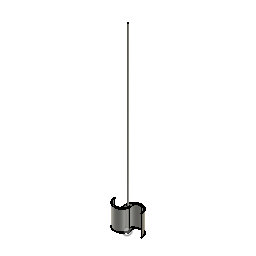
Savonius Turbine (Autodesk Fusion 360 design; units mm, degrees)
Autodesk Fusion 360 part; units mm, degrees
note: some values were not read from the file. Set by a fixed rule: which face or edge a step refers to.
sketch "Turbine Blade" plane through (0, 0, 0) normal (0, 0, 1) x (1, 0, 0) in component "Savonius Turbine"
  circle A0 centre (0, 0) radius 10.5 construction
  line L0 (0, 0) -> (-10.5, 0) construction
  line L1 (-10.5, 0) -> (75, 0) construction
  arc A1 (75, 0) -> (-10.5, 0) centre (32.25, 0) ccw
  arc A2 (74.2, 0) -> (-9.7, 0) centre (32.25, 0) ccw
  line L2 (74.2, 0) -> (75, 0)
  line L3 (-10.5, 0) -> (-9.7, 0) construction
  line L4 (-9.7, 0) -> (-10.5, 0)
  line L5 (75, 0) -> (37.5, 0)
  arc A3 (74.2, 0) -> (37.5, 36.7) centre (37.5, 0) ccw
  line L6 (37.5, 0) -> (74.2, 0) construction
  line L7 (37.5, 0) -> (37.5, 36.7) construction
  line L8 (37.5, 36.7) -> (0, 36.7) construction
  line L9 (0, 36.7) -> (-9.7, 0) construction
  spline S0 degree 2 poles (37.5, 36.7) (0, 36.7) (-9.7, 0) knots 0 0 0 1 1 1
  dimension "d57" = 21
  dimension "d59" = 75
  dimension "d84" = 42.75
  dimension "d87" = 37.5
  dimension "d88" = 90
  constraint coincident A0.centre L0.start
  constraint coincident A0 L0.end
  constraint horizontal L0
  constraint horizontal L1
  constraint parallel L1 L2
  constraint parallel L1 L3
  constraint coincident L1 L5.end
  constraint coincident L5.end A3.centre
  constraint horizontal L8
  constraint vertical A0.centre L8.end
  measures "d57" diameter of A0
  measures "d59" distance of L1.end A0.centre
  measures "d84" radius of A1
  measures "d87" distance of L1.end L5.end
  measures "d88" angle of L6 L7
extrude "Extrude5" add sketch "Turbine Blade" along normal blind 115.5 makes body 1 in component "Savonius Turbine"
pattern_circular "C-Pattern1" count 2 over 360 about axis through (0, 0, 1.75) along (0, 0, 1) of bodies 1 makes body 2 in component "Savonius Turbine"
sketch "EndPlates" plane through (0, 0, 0) normal (0, 0, 1) x (1, 0, 0) in component "Savonius Turbine"
  circle A0 centre (0, 0) radius 82.5
  line L0 (7.4921, 18.5437) -> (-7.4921, -18.5437) construction
  circle A1 centre (7.4921, 18.5437) radius 1.5
  circle A2 centre (-7.4921, -18.5437) radius 1.5
  line L1 (20, 0) -> (2.5, 0)
  circle A3 centre (0, 0) radius 4.25
  arc A4 (75, 0) -> (-10.5, 0) centre (32.25, 0) ccw
  line L2 (-10.5, 0) -> (-9.7, 0)
  spline S0 degree 2 poles (-9.7, 0) (0, 36.7) (37.5, 36.7) knots -1 -1 -1 0 0 0
  arc A5 (74.2, 0) -> (37.5, 36.7) centre (37.5, 0) ccw
  line L3 (74.2, 0) -> (75, 0)
  arc A6 (-75, 0) -> (10.5, 0) centre (-32.25, 0) ccw
  line L4 (10.5, 0) -> (9.7, 0)
  spline S1 degree 2 poles (9.7, 0) (0, -36.7) (-37.5, -36.7) knots -1 -1 -1 0 0 0
  arc A7 (-74.2, 0) -> (-37.5, -36.7) centre (-37.5, 0) ccw
  line L5 (-74.2, 0) -> (-75, 0)
  arc A8 (-72.1423, 2) -> (-37.5, -34.7) centre (-37.5, 0) ccw
  spline S2 degree 3 poles (8.1599, 2) (8.0288, 1.5037) (7.8976, 1.0074) (7.7664, 0.5111) (4.8101, -10.674) (-0.0689, -19.0509) (-6.813, -24.8318) (-13.502, -30.5653) (-22.0851, -33.8174) (-32.8116, -34.5451) (-34.332, -34.6482) (-35.8948, -34.7) (-37.5, -34.7) knots -1.020285 -1.020285 -1.020285 -1.020285 -1 -1 -1 -0.531046 -0.531046 -0.531046 -0.065928 -0.065928 -0.065928 0 0 0 0
  line L6 (12.4553, 2) -> (8.1599, 2)
  arc A9 (-76.9553, 2) -> (12.4553, 2) centre (-32.25, 0) ccw
  line L7 (-72.1423, 2) -> (-76.9553, 2)
  arc A10 (72.1423, -2) -> (37.5, 34.7) centre (37.5, 0) ccw
  spline S3 degree 3 poles (-8.1599, -2) (-8.0288, -1.5037) (-7.8976, -1.0074) (-7.7664, -0.5111) (-4.8101, 10.674) (0.0689, 19.0509) (6.813, 24.8318) (13.502, 30.5653) (22.0851, 33.8174) (32.8116, 34.5451) (34.332, 34.6482) (35.8948, 34.7) (37.5, 34.7) knots -1.020285 -1.020285 -1.020285 -1.020285 -1 -1 -1 -0.531046 -0.531046 -0.531046 -0.065928 -0.065928 -0.065928 0 0 0 0
  line L8 (-12.4553, -2) -> (-8.1599, -2)
  arc A11 (76.9553, -2) -> (-12.4553, -2) centre (32.25, 0) ccw
  line L9 (72.1423, -2) -> (76.9553, -2)
  line L10 (-12.4553, -2) -> (-11.2868, -28.1194)
  line L11 (12.4553, 2) -> (11.2868, 28.1194)
  dimension "d65" = 165
  dimension "d68" = 40
  dimension "d69" = 3
  dimension "d70" = 3
  dimension "d71" = 68
  dimension "d72" = 8.5
  dimension "d89" = 2
  dimension "d90" = 2
  constraint coincident A0.centre A3.centre
  constraint midpoint L0 A0.centre
  constraint coincident L0.start A1.centre
  constraint coincident L0.end A2.centre
  constraint concentric A0 A3
  constraint coincident S2 L10.end
  constraint tangent A11 L10
  constraint coincident S3 L11.end
  constraint tangent A9 L11
  measures "d65" diameter of A0
  measures "d68" distance of L0.start L0.end
  measures "d69" diameter of A1
  measures "d70" diameter of A2
  measures "d71" angle of L0 L1
  measures "d72" diameter of A3
extrude "Extrude6" add sketch "EndPlates" along normal blind 2.4 separate body contours L1 A6 L4 S1 A7 L5 | L1 L4 S2 L6 A9 | L1 A6 S1 A7 L5 A8 S2 A9 L7 | S2 L6 S3 L8 L10 L11 | A10 S3 L8 A11 L9 | A4 L2 S0 A5 L3 makes body 3 in component "Savonius Turbine"
extrude "Extrude7" add sketch "EndPlates" along normal mid plane 2.4 from surface at 115.5 separate body contours L1 A6 L4 S1 A7 L5 | L1 L4 S2 L6 A9 | L1 A6 S1 A7 L5 A8 S2 A9 L7 | S2 L6 S3 L8 L10 L11 | A10 S3 L8 A11 L9 | A4 L2 S0 A5 L3 makes body 4 in component "Savonius Turbine"
combine "Combine1" operation cut target body 4 tool bodies 1 2 keep tools in component "Savonius Turbine"
combine "Combine2" operation add target body 3 tool bodies 2 1 in component "Savonius Turbine"
move_face "OffsetFaces1" offset -0.1 10 faces at (64.9984, 27.4792, 114.7) (74.0338, 3.4886, 114.7) (-8.2372, 4.8659, 114.7) (-9.9667, 0, 114.7) (74.4667, 0, 114.7) (-64.9984, -27.4792, 114.7) (-74.0338, -3.4886, 114.7) (8.2372, -4.8659, 114.7) (9.9667, 0, 114.7) (-74.4667, 0, 114.7) on bodies 4 in component "Savonius Turbine"
chamfer "Chamfer1" distance 1.9 angle 45 10 edges at (-63.4508, -25.9508, 2.4) (-6.8878, -27.4766, 2.4) (32.25, 42.75, 2.4) (63.4508, 25.9508, 2.4) (6.8878, 27.4766, 2.4) (-32.25, -42.75, 2.4) (74.6, 0, 2.4) (-74.6, 0, 2.4) (-10.1, 0, 2.4) (10.1, 0, 2.4) on bodies 3 in component "Savonius Turbine"
move_face "OffsetFaces2" offset 1.9 1 faces at (7.7745, 7.3191, 114.3) on bodies 4 in component "Savonius Turbine"
chamfer "Chamfer2" distance 1.89 angle 45 10 edges at (-32.25, -44.75, 112.4) (11.871, 15.0597, 112.4) (23.8531, 33.2388, 112.4) (62.7338, 23.819, 112.4) (74.5488, -2, 112.4) (32.25, 44.75, 112.4) (-11.871, -15.0597, 112.4) (-62.7338, -23.819, 112.4) (-23.8531, -33.2388, 112.4) (-74.5488, 2, 112.4) on bodies 4 in component "Savonius Turbine"
cylinder "CylinderPrimitive1" add diameter 8 height 1000 placed x (1, 0, 0) y (0, 1, 0) z (0, 0, 1) at (0, 0, 0) separate body makes body 5 in component "Shaft"
sketch "Sketch1" plane through (0, 0, 0) normal (0, 0, 1) x (1, 0, 0) in component "Shaft grippy thing"
  circle A0 centre (0, 0) radius 4
  circle A1 centre (0, 0) radius 6
  circle A2 centre (0, 0) radius 4.3
  dimension "d97" = 12
  dimension "d98" = 8.6
  constraint concentric A0 A1
  constraint concentric A1 A2
  measures "d97" diameter of A1
  measures "d98" diameter of A2
extrude "Extrude1" add sketch "Sketch1" along normal blind 12 separate body contours A2 makes body 6 in component "Shaft grippy thing"
extrude "Extrude2" add sketch "Sketch1" along normal blind 7 contours A1 bodies 6 in component "Shaft grippy thing"
ref_plane "WorkPlane1" through (-6, 0, 4.0759) normal (-1, 0, 0) x (0, 1, 0) in component "Shaft grippy thing"
sketch "Sketch2" plane through (-6, 0, 0) normal (-1, 0, 0) x (0, -1, 0) in component "Shaft grippy thing"
  line L0 (6, 7) -> (-6, 7)
  line L1 (6, 0) -> (-6, 0)
  line L2 (0, 0) -> (0, 4.9977) construction
  line L3 (0.5, 0) -> (0.5, 8)
  line L4 (-0.5, 0) -> (-0.5, 8)
  line L5 (0.5, 8) -> (0, 8.866)
  line L6 (-0.5, 8) -> (0, 8.866)
  line L7 (-2.75, 6) -> (2.75, 6)
  line L8 (2.75, 6) -> (2.75, 0)
  line L9 (2.75, 0) -> (-2.75, 0)
  line L10 (-2.75, 0) -> (-2.75, 6)
  line L11 (-2.75, 6) -> (2.75, 0) construction
  line L12 (2.75, 6) -> (-2.75, 0) construction
  point P0 (0, 3)
  dimension "d104" = 60
  dimension "d105" = 5.5
  dimension "d106" = 6
  dimension "d107" = 1
  dimension "d108" = 1
  constraint coincident L2.start origin
  constraint perpendicular L1 L2
  constraint coincident L1 L3.start
  constraint perpendicular L1 L3
  constraint symmetric L2 L3.start L4.start
  constraint symmetric L2 L3.end L4.end
  constraint horizontal L7
  constraint perpendicular L7 L8
  constraint parallel L7 L9
  constraint parallel L8 L10
  constraint coincident L11 P0
  constraint coincident L12 P0
  constraint coincident L2 P0
  constraint collinear L1 L9
  measures "d104" angle of L5 L6
  measures "d105" distance of L8.end L9.end
  measures "d106" distance of L7.end L8.end
  measures "d107" distance of L3 L4
  measures "d108" distance of L0 L4.end
extrude "Extrude1'" [suppressed] in component "Shaft"
extrude "Extrude3" cut sketch "Sketch2" against normal blind 2.0314 contours L0 L3 L4 L7 | L0 L3 L4 L5 L6 | L1 L3 L4 L7 L9 bodies 6 in component "Shaft grippy thing"
extrude "Extrude4" add sketch "Sketch2" along normal blind 5 and the other way up to surface contours L1 L3 L7 L8 L9 | L1 L4 L7 L9 L10 second end surface at (-3.8273, 4.6208, 2.3333) on bodies 6 bodies 6 in component "Shaft grippy thing"
sketch "Sketch3" plane through (0, 2.75, 0) normal (0, 1, 0) x (-1, 0, 0) in component "Shaft grippy thing"
  line L0 (5.3327, 0) -> (11, 0)
  line L1 (11, 0) -> (11, 6)
  line L2 (11, 6) -> (5.3327, 6)
  line L3 (5.3327, 6) -> (5.3327, 0)
  line L4 (8.1663, 6) -> (8.1663, 3) construction
  constraint midpoint L2 L4.start
  constraint perpendicular L2 L4
hole "Hole1" at (-8.1663, 2.75, 3) direction (0, -1, 0) diameter 3.1 depth 8.334 tip angle 118 bodies 6 in component "Shaft grippy thing"
chamfer "Chamfer1'" distance 1 angle 45 2 edges at (-5.7667, 1.6568, 6) (-5.7667, -1.6568, 6) on bodies 6 in component "Shaft grippy thing"
move_body "Move1" bodies 3 4 to x (1, 0, 0) y (0, 1, 0) z (0, 0, 1) at (0, 0, 12.782) in component "Savonius Turbine"
copy_body "Body->Comp1" bodies 4 removing the originals makes body 7 in component "Mini-Top"
component "Savonius Turbine" placed x (1, 0, 0) y (0, 1, 0) z (0, 0, 1) at (0, 0, 0)
component "Shaft" placed x (1, 0, 0) y (0, 1, 0) z (0, 0, 1) at (0, 0, 0)
component "Mini-Top" placed x (1, 0, 0) y (0, 1, 0) z (0, 0, 1) at (0, 0, 0) in component "Savonius Turbine"
component "Shaft grippy thing" placed x (1, 0, 0) y (0, 1, 0) z (0, 0, 1) at (0, 0, 0) in component "Shaft"
equation "Width = 150 mm" comment "Width of the turbine"
equation "AspectRatio = 0.77"
equation "OverlapPercent = 0.14" comment "How far the blades should overlap.  e.g. 0.10 would be 10%"
equation "Height = Width * AspectRatio"
equation "Overlap = OverlapPercent * Width"
equation "BladeDiameter = ( Width + Overlap ) / 2"
equation "BladeThickness = 0.8 mm"
equation "BaseThickness = 2.4 mm"
equation "Twist = 0.5"
equation "NumberOfBlades = 2"
equation "d57 = Overlap"
equation "d59 = Width / 2"
equation "d60 = -BladeThickness"
equation "d61 = Height"
equation "d63 = NumberOfBlades"
equation "d65 = Width * BaseRatio"
equation "d66 = BaseThickness"
equation "d73 = Height"
equation "d74 = BaseThickness"
equation "BaseRatio = 1.1" comment "This is the ratio of the diameter of the end plates to the width.  e.g. 1.1 means the end plates are 10% larger than the width"
equation "d87 = d59 / 2"
named bodies: "Blade1", "Blade2", "Mini-Top", "Bottom", "Shaft", "Shaft grippy thing"
